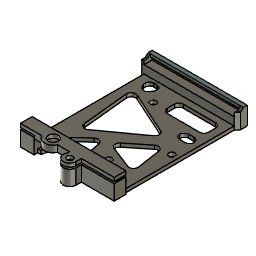
MCU_PCB_mount v14 (Autodesk Fusion 360 design; units mm, degrees)
Autodesk Fusion 360 part; units mm, degrees
sketch "Sketch1" plane through (0, 0, 0) normal (0, 0, 1) x (1, 0, 0)
  line L0 (0, 0) -> (50.2, 0)
  line L1 (50.2, 0) -> (50.2, 70.11)
  line L2 (50.2, 70.11) -> (0, 70.11)
  line L3 (0, 70.11) -> (0, 0)
  dimension "d3" = 50.2
  dimension "d4" = 70.11
  constraint horizontal L0
  constraint vertical L1
  constraint horizontal L2
  constraint vertical L3
  constraint coincident L0.start L3.end
  measures "d3" distance of L1.end L2.end
  measures "d4" distance of L0.end L1.end
extrude "Extrude1" add sketch "Sketch1" along normal blind 2 makes body 1
sketch "holes" plane through (0, 0, 2) normal (0, 0, 1) x (-1, 0, 0)
  line L0 (0, -70.11) -> (0, 0)
  line L1 (0, 0) -> (-50.2, 0)
  line L2 (-50.2, 0) -> (-50.2, -70.11)
  line L3 (-50.2, -70.11) -> (0, -70.11)
  line L4 (-14.9, 0) -> (-14.9, -55.81) construction
  line L5 (-14.9, -55.81) -> (-50.2, -55.81) construction
  line L6 (-48.02, -55.81) -> (-48.02, 0) construction
  line L7 (-16.3, -54.41) -> (-21.3533, -54.41) construction
  line L8 (-21.3533, -54.41) -> (-26.4067, -54.41) construction
  line L9 (-26.4067, -54.41) -> (-31.46, -54.41) construction
  line L10 (-31.46, -54.41) -> (-36.5133, -54.41) construction
  line L11 (-36.5133, -54.41) -> (-41.5667, -54.41) construction
  line L12 (-41.5667, -54.41) -> (-46.62, -54.41) construction
  circle A0 centre (-16.3, -54.41) radius 1.5 construction
  circle A1 centre (-21.3533, -54.41) radius 1.5 construction
  circle A2 centre (-26.4067, -54.41) radius 1.5 construction
  circle A3 centre (-31.46, -54.41) radius 1.5 construction
  circle A4 centre (-36.5133, -54.41) radius 1.5 construction
  circle A5 centre (-41.5667, -54.41) radius 1.5 construction
  circle A6 centre (-46.62, -54.41) radius 1.5 construction
  line L13 (-14.9, -55.81) -> (-17.7, -55.81) construction
  line L14 (-17.7, -55.81) -> (-17.7, -53.01) construction
  line L15 (-17.7, -53.01) -> (-14.9, -53.01) construction
  line L16 (-14.9, -53.01) -> (-14.9, -55.81) construction
  line L17 (-14.9, -55.81) -> (-17.7, -53.01) construction
  line L18 (-17.7, -55.81) -> (-14.9, -53.01) construction
  line L19 (-16.3, -54.41) -> (-14.9, -54.41) construction
  line L20 (-46.62, -54.41) -> (-48.02, -54.41) construction
  circle A7 centre (-16.3, -49.437) radius 1.5 construction
  circle A8 centre (-21.3533, -49.437) radius 1.5 construction
  circle A9 centre (-26.4067, -49.437) radius 1.5 construction
  circle A10 centre (-31.46, -49.437) radius 1.5 construction
  circle A11 centre (-36.5133, -49.437) radius 1.5 construction
  circle A12 centre (-41.5667, -49.437) radius 1.5 construction
  circle A13 centre (-46.62, -49.437) radius 1.5 construction
  circle A14 centre (-16.3, -44.464) radius 1.5 construction
  circle A15 centre (-21.3533, -44.464) radius 1.5 construction
  circle A16 centre (-26.4067, -44.464) radius 1.5 construction
  circle A17 centre (-31.46, -44.464) radius 1.5 construction
  circle A18 centre (-36.5133, -44.464) radius 1.5 construction
  circle A19 centre (-41.5667, -44.464) radius 1.5 construction
  circle A20 centre (-46.62, -44.464) radius 1.5 construction
  circle A21 centre (-16.3, -39.491) radius 1.5 construction
  circle A22 centre (-21.3533, -39.491) radius 1.5 construction
  circle A23 centre (-26.4067, -39.491) radius 1.5 construction
  circle A24 centre (-31.46, -39.491) radius 1.5 construction
  circle A25 centre (-36.5133, -39.491) radius 1.5 construction
  circle A26 centre (-41.5667, -39.491) radius 1.5 construction
  circle A27 centre (-46.62, -39.491) radius 1.5 construction
  circle A28 centre (-16.3, -34.518) radius 1.5 construction
  circle A29 centre (-21.3533, -34.518) radius 1.5 construction
  circle A30 centre (-26.4067, -34.518) radius 1.5 construction
  circle A31 centre (-31.46, -34.518) radius 1.5 construction
  circle A32 centre (-36.5133, -34.518) radius 1.5 construction
  circle A33 centre (-41.5667, -34.518) radius 1.5 construction
  circle A34 centre (-46.62, -34.518) radius 1.5 construction
  circle A35 centre (-16.3, -29.545) radius 1.5 construction
  circle A36 centre (-21.3533, -29.545) radius 1.5 construction
  circle A37 centre (-26.4067, -29.545) radius 1.5 construction
  circle A38 centre (-31.46, -29.545) radius 1.5 construction
  circle A39 centre (-36.5133, -29.545) radius 1.5 construction
  circle A40 centre (-41.5667, -29.545) radius 1.5 construction
  circle A41 centre (-46.62, -29.545) radius 1.5 construction
  circle A42 centre (-16.3, -24.572) radius 1.5 construction
  circle A43 centre (-21.3533, -24.572) radius 1.5 construction
  circle A44 centre (-26.4067, -24.572) radius 1.5 construction
  circle A45 centre (-31.46, -24.572) radius 1.5 construction
  circle A46 centre (-36.5133, -24.572) radius 1.5 construction
  circle A47 centre (-41.5667, -24.572) radius 1.5 construction
  circle A48 centre (-46.62, -24.572) radius 1.5 construction
  circle A49 centre (-16.3, -19.599) radius 1.5 construction
  circle A50 centre (-21.3533, -19.599) radius 1.5 construction
  circle A51 centre (-26.4067, -19.599) radius 1.5 construction
  circle A52 centre (-31.46, -19.599) radius 1.5 construction
  circle A53 centre (-36.5133, -19.599) radius 1.5 construction
  circle A54 centre (-41.5667, -19.599) radius 1.5 construction
  circle A55 centre (-46.62, -19.599) radius 1.5 construction
  circle A56 centre (-16.3, -14.626) radius 1.5 construction
  circle A57 centre (-21.3533, -14.626) radius 1.5 construction
  circle A58 centre (-26.4067, -14.626) radius 1.5 construction
  circle A59 centre (-31.46, -14.626) radius 1.5 construction
  circle A60 centre (-36.5133, -14.626) radius 1.5 construction
  circle A61 centre (-41.5667, -14.626) radius 1.5 construction
  circle A62 centre (-46.62, -14.626) radius 1.5 construction
  circle A63 centre (-16.3, -9.653) radius 1.5 construction
  circle A64 centre (-21.3533, -9.653) radius 1.5 construction
  circle A65 centre (-26.4067, -9.653) radius 1.5 construction
  circle A66 centre (-31.46, -9.653) radius 1.5 construction
  circle A67 centre (-36.5133, -9.653) radius 1.5 construction
  circle A68 centre (-41.5667, -9.653) radius 1.5 construction
  circle A69 centre (-46.62, -9.653) radius 1.5 construction
  circle A70 centre (-16.3, -4.68) radius 1.5 construction
  circle A71 centre (-21.3533, -4.68) radius 1.5 construction
  circle A72 centre (-26.4067, -4.68) radius 1.5 construction
  circle A73 centre (-31.46, -4.68) radius 1.5 construction
  circle A74 centre (-36.5133, -4.68) radius 1.5 construction
  circle A75 centre (-41.5667, -4.68) radius 1.5 construction
  circle A76 centre (-46.62, -4.68) radius 1.5 construction
  line L21 (-14.9, -3.27) -> (-48.02, -3.27) construction
  line L22 (-16.3, -3.27) -> (-16.3, -4.67) construction
  line L23 (-16.3, -54.41) -> (-16.3, -55.81) construction
  point P0 (-16.3, -54.41)
  dimension "d8" = 14.9
  dimension "d9" = 14.3
  dimension "d10" = 2.18
  dimension "d13" = 3
  dimension "d14" = 2.8
  dimension "d15" = 5.0533
  dimension "d18" = 0
  dimension "d19" = 49.73
  dimension "d40" = 52.54
  constraint coincident L1 L4.start
  constraint perpendicular L1 L4
  constraint coincident L2 L5.end
  constraint perpendicular L2 L5
  constraint coincident L5 L6.start
  constraint coincident L1 L6.end
  constraint perpendicular L1 L6
  constraint perpendicular L4 L7
  constraint perpendicular L4 L8
  constraint parallel L8 L9
  constraint parallel L9 L10
  constraint parallel L10 L11
  constraint parallel L11 L12
  constraint equal L7 L8
  constraint equal L8 L9
  constraint equal L9 L10
  constraint equal L10 L11
  constraint equal L11 L12
  constraint coincident P0 L7.start
  constraint coincident L7.end L8.start
  constraint coincident L8.end L9.start
  constraint coincident L9.end L10.start
  constraint coincident L10.end L11.start
  constraint coincident L11.end L12.start
  constraint coincident L12.end A6.centre
  constraint equal A0 A1
  constraint equal A1 A2
  constraint equal A2 A3
  constraint equal A3 A4
  constraint equal A4 A5
  constraint equal A5 A6
  constraint horizontal L13
  constraint perpendicular L13 L14
  constraint parallel L13 L15
  constraint parallel L14 L16
  constraint coincident L17 P0
  constraint coincident L18 P0
  constraint equal L14 L15
  constraint midpoint L16 L19.end
  constraint coincident L6 L20.end
  constraint perpendicular L6 L20
  constraint equal L19 L20
  constraint coincident L4 L21.start
  constraint coincident L6 L21.end
  constraint perpendicular L6 L21
  constraint coincident L21 L22.start
  constraint perpendicular L21 L22
  constraint midpoint L13 L23.end
  constraint equal L22 L23
  constraint vertical A70.centre L22.end
  measures "d8" distance of L0 L4
  measures "d9" distance of L3 L5
  measures "d10" distance of L2 L6
  measures "d13" diameter of A0
  measures "d14" distance of L13.end L14.end
  measures "d15" distance of P0 L7.end
  measures "d40" distance of L5 L21
sketch "screw-around" plane through (0, 0, 2) normal (0, 0, 1) x (-1, 0, 0)
  line L0 (0, -70.11) -> (0, 0)
  line L1 (0, 0) -> (-50.2, 0)
  line L2 (-50.2, 0) -> (-50.2, -70.11)
  line L3 (-50.2, -70.11) -> (0, -70.11)
  line L4 (-15.1, -3.845) -> (-15.1, 3.845) construction
  circle A0 centre (-15.1, 0) radius 3.845 construction
  dimension "d68" = 15.1
  dimension "d69" = 7.69
  constraint perpendicular L1 L4
  constraint coincident L4 A0.centre
  constraint coincident L1 A0.centre
  constraint coincident L4.start A0
  constraint coincident L4.end A0
  measures "d68" distance of L0 L4
  measures "d69" diameter of A0
sketch "Sketch7" plane through (0, 0, 2) normal (0, 0, 1) x (-1, 0, 0)
  line L0 (0, -70.11) -> (0, 0)
  line L1 (0, 0) -> (-50.2, 0)
  line L2 (-50.2, 0) -> (-50.2, -70.11)
  line L3 (-50.2, -70.11) -> (0, -70.11)
  circle A0 centre (-16.3, -54.41) radius 1.5
  circle A1 centre (-31.46, -4.68) radius 1.5
  circle A2 centre (-46.62, -34.518) radius 1.5
  circle A3 centre (-31.46, -14.626) radius 1.5
extrude "Extrude6" cut sketch "Sketch7" against normal up to surface (2 mm away) contours A0 | A2 | A3 bodies 1
sketch "Sketch8" plane through (0, 0, 0) normal (0, 0, 1) x (1, 0, 0)
  line L0 (-1.6, 65.61) -> (51.8, 65.61)
  line L1 (51.8, 65.61) -> (51.8, 71.71)
  line L2 (51.8, 71.71) -> (-1.6, 71.71)
  line L3 (-1.6, 71.71) -> (-1.6, 65.61)
  line L4 (50.2, 70.11) -> (0, 70.11)
  line L5 (0, 70.11) -> (0, 0) construction
  line L6 (50.2, 0) -> (50.2, 70.11) construction
  dimension "d45" = 4.5
  dimension "d46" = 1.6
  dimension "d47" = 1.6
  dimension "d48" = 1.6
  constraint horizontal L0
  constraint vertical L1
  constraint horizontal L2
  constraint vertical L3
  measures "d45" distance of L0 L4
  measures "d46" distance of L2 L4
  measures "d47" distance of L3 L5
  measures "d48" distance of L1 L6
extrude "Extrude7" add sketch "Sketch8" along normal blind 6.5 bodies 1
sketch "Sketch9" plane through (0, 0, 6.5) normal (0, 0, 1) x (-1, 0, 0)
  line L0 (1.6, -71.71) -> (1.6, -65.61)
  line L1 (1.6, -65.61) -> (-51.8, -65.61)
  line L2 (-51.8, -65.61) -> (-51.8, -71.71)
  line L3 (-51.8, -71.71) -> (1.6, -71.71)
  line L4 (0, -65.61) -> (-50.2, -65.61)
  line L5 (-50.2, -65.61) -> (-50.2, -70.11)
  line L6 (-50.2, -70.11) -> (0, -70.11)
  line L7 (0, -70.11) -> (0, -65.61)
  line L8 (0, -65.61) -> (0, 0)
  line L9 (-50.2, 0) -> (-50.2, -65.61)
  dimension "d51" = 1.6
  constraint horizontal L4
  constraint vertical L5
  constraint horizontal L6
  constraint vertical L7
  constraint coincident L1 L4.start
  constraint collinear L7 L8
  constraint collinear L5 L9
  measures "d51" distance of L3 L6
extrude "Extrude8" add sketch "Sketch9" along normal blind 1.9 contours L0 L1 L2 L3 L5 L6 L7 bodies 1
sketch "Sketch10" plane through (0, 0, 8.4) normal (0, 0, 1) x (-1, 0, 0)
  line L0 (-50.2, -65.61) -> (-51.8, -65.61)
  line L1 (-51.8, -65.61) -> (-51.8, -71.71)
  line L2 (-51.8, -71.71) -> (1.6, -71.71)
  line L3 (1.6, -71.71) -> (1.6, -65.61)
  line L4 (1.6, -65.61) -> (0, -65.61)
  line L5 (0, -65.61) -> (0, -70.11)
  line L6 (0, -70.11) -> (-50.2, -70.11)
  line L7 (-50.2, -70.11) -> (-50.2, -65.61)
  line L8 (1.6, -71.71) -> (-51.8, -71.71)
  line L9 (-51.8, -71.71) -> (-51.8, -69.11)
  line L10 (-51.8, -69.11) -> (1.6, -69.11)
  line L11 (1.6, -69.11) -> (1.6, -71.71)
  dimension "d56" = 1
  constraint horizontal L8
  constraint vertical L9
  constraint horizontal L10
  constraint vertical L11
  constraint coincident L1 L9.end
  constraint coincident L2.end L3.start
  measures "d56" distance of L6 L10
extrude "Extrude9" add sketch "Sketch10" along normal blind 1.6 contours L5 L6 L7 L10 | L1 L2 L3 L5 L6 L7 L8 L9 L10 L11 bodies 1
chamfer "Chamfer1" distance 1.6 angle 45 2 edges at (-0.8, 69.11, 8.4) (51, 69.11, 8.4) on bodies 1
sketch "Sketch11" plane through (0, 0, 0) normal (0, 0, 1) x (1, 0, 0)
  line L0 (-1.6, 4.5) -> (51.8, 4.5)
  line L1 (51.8, 4.5) -> (51.8, -2)
  line L2 (51.8, -2) -> (-1.6, -2)
  line L3 (-1.6, -2) -> (-1.6, 4.5)
  line L4 (0, 0) -> (50.2, 0)
  line L5 (6.4, 4.5) -> (6.4, -2)
  line L6 (27.8, 4.5) -> (27.8, -2)
  point P0 (-1.6, 65.61)
  point P1 (51.8, 65.61)
  dimension "d60" = 2
  dimension "d61" = 4.5
  dimension "d62" = 24
  dimension "d63" = 8
  constraint horizontal L0
  constraint vertical L1
  constraint horizontal L2
  constraint vertical L3
  constraint vertical L0.start P0
  constraint vertical L0.end P1
  constraint coincident L0 L5.start
  constraint coincident L2 L5.end
  constraint perpendicular L2 L5
  constraint coincident L0 L6.start
  constraint coincident L2 L6.end
  constraint perpendicular L2 L6
  measures "d60" distance of L2 L4
  measures "d61" distance of L0 L4
  measures "d62" distance of L1 L6
  measures "d63" distance of L3 L5
extrude "Extrude10" add sketch "Sketch11" along normal up to surface (8.4 mm away) contours L0 L2 L3 L5 | L0 L1 L2 L6 bodies 1
sketch "Sketch12" plane through (0, 0, 8.4) normal (0, 0, 1) x (-1, 0, 0)
  line L0 (-6.4, 2) -> (-6.4, -4.5)
  line L1 (-6.4, -4.5) -> (1.6, -4.5)
  line L2 (1.6, -4.5) -> (1.6, 2)
  line L3 (1.6, 2) -> (-6.4, 2)
  line L4 (0, 0.4) -> (-50.2, 0.4)
  line L5 (-50.2, 0.4) -> (-50.2, -4.5)
  line L6 (-50.2, -4.5) -> (0, -4.5)
  line L7 (0, -4.5) -> (0, 0.4)
  line L8 (-50.2, -4.5) -> (-50.2, -65.61)
  line L9 (0, -65.61) -> (0, -4.5)
  line L10 (-6.4, 0) -> (-27.8, 0) construction
  dimension "d80" = 0.4
  constraint horizontal L4
  constraint vertical L5
  constraint horizontal L6
  constraint vertical L7
  constraint collinear L5 L8
  constraint collinear L1 L6
  constraint coincident L4.end L5.start
  constraint collinear L7 L9
  measures "d80" distance of L4 L10
extrude "Extrude11" cut sketch "Sketch12" against normal up to surface (1.9 mm away) contours L0 L1 L4 L6 L7 | L0 L4 L5 L6 bodies 1
sketch "Sketch14" plane through (0, 0, 2) normal (0, 0, 1) x (-1, 0, 0)
  line L0 (-27.8, -4.5) -> (-50.2, -4.5)
  line L1 (-50.2, -4.5) -> (-50.2, -65.61)
  line L2 (-50.2, -65.61) -> (0, -65.61)
  line L3 (0, -65.61) -> (0, -4.5)
  line L4 (0, -4.5) -> (-6.4, -4.5)
  line L5 (-6.4, -4.5) -> (-6.4, 0)
  line L6 (-6.4, 0) -> (-27.8, 0)
  line L7 (-27.8, 0) -> (-27.8, -4.5)
  circle A0 centre (-16.3, -54.41) radius 1.5
  circle A1 centre (-46.62, -34.518) radius 1.5
  circle A2 centre (-31.46, -14.626) radius 1.5
  circle A3 centre (-15.1, 0) radius 3.845 construction
  circle A4 centre (-15.1, 0) radius 6.845
  dimension "d70" = 3
  constraint concentric A3 A4
  measures "d70" distance of A3 A4
extrude "Extrude12" cut sketch "Sketch14" against normal up to surface (2 mm away) contours L6 A4 picked at (-15.9336, -2.8041) bodies 1
sketch "Sketch15" plane through (0, 0, 0) normal (0, 0, 1) x (1, 0, 0)
  circle A0 centre (29.2, -5) radius 1.5
  circle A1 centre (29.2, -5) radius 3.5
  line L0 (21.945, 0) -> (27.8, 0)
  line L1 (50.2, 4.5) -> (50.2, -0.4)
  line L2 (32.7, -5) -> (32.7, -0.4)
  line L3 (26.1623, -3.2615) -> (27.8, -0.4)
  line L4 (27.8, -0.4) -> (32.7, -0.4)
  point P0 (27.8, -0.4)
  dimension "d73" = 3
  dimension "d74" = 2
  dimension "d76" = 5
  dimension "d77" = 21
  constraint concentric A0 A1
  constraint coincident A1 L2.start
  constraint perpendicular L0 L2
  constraint tangent A1 L2
  constraint coincident A1 L3.start
  constraint coincident P0 L3.end
  constraint tangent A1 L3
  constraint perpendicular L2 L4
  measures "d73" diameter of A0
  measures "d74" distance of A0 A1
  measures "d76" distance of A0.centre L0
  measures "d77" distance of A0.centre L1
extrude "Extrude13" add sketch "Sketch15" along normal up to surface (8.4 mm away) bodies 1
fillet "Fillet1" radius 15.75 1 edges at (27.8, -0.4, 3.25) on bodies 1
fillet "Fillet2" radius 2 1 edges at (27.3488, 0, 1) on bodies 1
sketch "cuts" plane through (0, 0, 2) normal (0, 0, 1) x (-1, 0, 0)
  arc A0 (-26.3604, 2.8353) -> (-27.8, -3.743) centre (-12.05, -3.743) ccw
  line L0 (-27.8, -3.743) -> (-27.8, -4.5)
  line L1 (-27.8, -4.5) -> (-50.2, -4.5)
  line L2 (-50.2, -4.5) -> (-50.2, -65.61)
  line L3 (-50.2, -65.61) -> (0, -65.61)
  line L4 (0, -65.61) -> (0, -4.5)
  line L5 (0, -4.5) -> (-6.4, -4.5)
  line L6 (-6.4, -4.5) -> (-6.4, 0)
  line L7 (-6.4, 0) -> (-8.255, 0)
  arc A1 (-21.945, 0) -> (-8.255, 0) centre (-15.1, 0) ccw
  line L8 (-21.945, 0) -> (-24.5432, 0)
  arc A2 (-26.3604, 2.8353) -> (-24.5432, 0) centre (-24.5432, 2) ccw
  circle A3 centre (-16.3, -54.41) radius 1.5
  circle A4 centre (-46.62, -34.518) radius 1.5
  circle A5 centre (-31.46, -14.626) radius 1.5
  line L9 (-36, -41) -> (-4.2679, -55.3205)
  line L10 (-4.2679, -55.3205) -> (-7.7321, -20.6795)
  line L11 (-7.7321, -20.6795) -> (-36, -41)
  line L12 (-44, -15) -> (-40.6603, -36.9282)
  line L13 (-40.6603, -36.9282) -> (-23.3397, -23.0718)
  line L14 (-23.3397, -23.0718) -> (-44, -15)
  line L15 (-23, -62) -> (-46, -62)
  line L16 (-46, -62) -> (-46, -53)
  line L17 (-46, -53) -> (-23, -53)
  line L18 (-23, -53) -> (-23, -62)
  line L19 (-39, -49) -> (-47, -49)
  line L20 (-47, -49) -> (-47, -44)
  line L21 (-47, -44) -> (-39, -44)
  line L22 (-39, -44) -> (-39, -49)
  line L23 (-37, -10) -> (-47, -10)
  line L24 (-47, -10) -> (-47, -6)
  line L25 (-47, -6) -> (-37, -6)
  line L26 (-37, -6) -> (-37, -10)
  line L27 (-20.2679, -23.6603) -> (-7, -12)
  line L28 (-7, -12) -> (-23.7321, -6.3397)
  line L29 (-23.7321, -6.3397) -> (-20.2679, -23.6603)
  line L30 (-2.8038, -64) -> (-8, -55)
  line L31 (-8, -55) -> (-13.1962, -64)
  line L32 (-13.1962, -64) -> (-2.8038, -64)
  point P0 (-16, -39)
  point P1 (-36, -25)
  point P2 (-17, -14)
  point P3 (-8, -61)
  constraint horizontal L15
  constraint vertical L16
  constraint horizontal L17
  constraint vertical L18
  constraint horizontal L19
  constraint vertical L20
  constraint horizontal L21
  constraint vertical L22
  constraint horizontal L23
  constraint vertical L24
  constraint horizontal L25
  constraint vertical L26
extrude "cuts" cut sketch "cuts" against normal up to surface (2 mm away) contours L9 L10 L11 | L12 L13 L14 | L15 L16 L17 L18 | L19 L20 L21 L22 | L23 L24 L25 L26 | L27 L28 L29 | L30 L31 L32 bodies 1
fillet "Fillet3" radius 2.5 24 edges at (36, 41, 1) (4.2679, 55.3205, 1) (7.7321, 20.6795, 1) (7, 12, 1) (20.2679, 23.6603, 1) (40.6603, 36.9282, 1) (47, 49, 1) (46, 62, 1) (23.7321, 6.3397, 1) (44, 15, 1) (47, 6, 1) (23.3397, 23.0718, 1) (37, 6, 1) (39, 44, 1) (23, 53, 1) (37, 10, 1) (47, 10, 1) (39, 49, 1) (23, 62, 1) (2.8038, 64, 1) (13.1962, 64, 1) (46, 53, 1) (47, 44, 1) (8, 55, 1) on bodies 1
ref_plane "WorkPlane1" through (38.3733, -2.3137, 9.4) normal (0, 0, 1) x (1, 0, 0)
sketch "Sketch17" plane through (38.5752, -2.3138, 9.4) normal (0, 0, 1) x (1, 0, 0)
  arc A0 (-12.4933, -1.0965) -> (-5.8752, -2.6862) centre (-9.3752, -2.6862) ccw construction
  line L0 (-10.7752, 6.8138) -> (11.6248, 6.8138) construction
  line L1 (13.2248, 6.8138) -> (13.2248, 0.3138) construction
  line L2 (-40.1752, 0.3138) -> (-40.1752, 6.8138) construction
  line L3 (13.2248, 0.3138) -> (-5.8752, 0.3138) construction
  circle A1 centre (-23.4752, 2.3138) radius 3.845 construction
  circle A2 centre (-9.3752, -2.6862) radius 3.5
  circle A3 centre (-9.3752, -2.6862) radius 1.7
  line L4 (-5.8752, -2.6862) -> (-5.8752, 0.3138)
  line L5 (-5.8752, 0.3138) -> (13.2248, 0.3138)
  line L6 (13.2248, 0.3138) -> (13.2248, 6.8138)
  line L7 (13.2248, 6.8138) -> (-40.1752, 6.8138)
  line L8 (-40.1752, 6.8138) -> (-40.1752, 0.3138)
  line L9 (-40.1752, 0.3138) -> (-27.8386, 0.3138)
  line L10 (-12.4933, -1.0965) -> (-12.4933, 0.3138)
  line L11 (-12.4933, 0.3138) -> (-19.1117, 0.3138)
  arc A4 (-27.8386, 0.3138) -> (-19.1117, 0.3138) centre (-23.4752, 2.3138) ccw
  circle A5 centre (-23.4752, 2.3138) radius 2.8
  dimension "d90" = 3.4
  dimension "d93" = 5.6
  dimension "d94" = 2
  constraint concentric A0 A2
  constraint coincident A0.end A2
  constraint concentric A0 A3
  constraint coincident A0.end L4.start
  constraint coincident L3.end L4.end
  constraint coincident L1.end L3.start
  constraint coincident L1.start L6.end
  constraint coincident L2.end L7.end
  constraint coincident L2.start L8.end
  constraint perpendicular L8 L9
  constraint coincident A0.start L10.start
  constraint vertical L10
  constraint perpendicular L10 L11
  constraint coincident A1.centre A4.centre
  constraint coincident L9.end A4.start
  constraint collinear L9 L11
  constraint concentric A4 A5
  measures "d90" diameter of A3
  measures "d93" diameter of A5
  measures "d94" distance of A4 A5
extrude "Extrude15" add sketch "Sketch17" along normal blind 2 separate body makes body 2
sketch "Sketch18" plane through (0, 0, 9.4) normal (0, 0, -1) x (1, 0, 0)
  circle A0 centre (29.2, 5) radius 1.7
  circle A1 centre (15.1, 0) radius 2.8
  arc A2 (32.7, 5) -> (26.0818, 3.4104) centre (29.2, 5) ccw
  line L0 (26.0818, 3.4104) -> (26.0818, 2)
  line L1 (26.0818, 2) -> (19.4635, 2)
  arc A3 (19.4635, 2) -> (10.7365, 2) centre (15.1, 0) ccw
  line L2 (10.7365, 2) -> (-1.6, 2)
  line L3 (-1.6, 2) -> (-1.6, -4.5)
  line L4 (-1.6, -4.5) -> (51.8, -4.5)
  line L5 (51.8, -4.5) -> (51.8, 2)
  line L6 (51.8, 2) -> (32.7, 2)
  line L7 (32.7, 2) -> (32.7, 5)
  line L8 (6.4, 0.4) -> (6.4, 2) construction
  arc A4 (27.2453, 0.4) -> (26.0818, 3.4104) centre (12.05, -3.743) ccw construction
  line L9 (26.0818, 2) -> (26.0818, 0.4)
  line L10 (26.0818, 0.4) -> (17.8713, 0.4)
  line L11 (6.8, 2) -> (6.8, 0.4)
  line L12 (6.8, 0.4) -> (12.3287, 0.4)
  line L13 (10.7365, 2) -> (19.4635, 2)
  circle A5 centre (15.1, 0) radius 2.8 construction
  arc A6 (13.6578, 2.4) -> (12.3287, 0.4) centre (15.1, 0) ccw
  arc A7 (17.8713, 0.4) -> (17.0596, 2) centre (15.1, 0) ccw
  dimension "d97" = 0.4
  constraint coincident L0.end L1.start
  constraint perpendicular L1 L9
  constraint coincident A1 L10.end
  constraint perpendicular L9 L10
  constraint coincident L2 L11.start
  constraint perpendicular L2 L11
  constraint coincident A1 L12.end
  constraint perpendicular L11 L12
  constraint collinear L10 L12
  constraint horizontal L8.start L11.end
  constraint coincident A3.end L2.start
  constraint coincident L1.end A3.start
  constraint equal A1 A5
  constraint concentric A1 A5
  constraint coincident A1.centre A3.centre
  constraint coincident A5 A7.end
  constraint coincident L13 A7.end
  measures "d97" distance of L8 L11
extrude "Extrude16" add sketch "Sketch18" along normal blind 1.7 contours A1 L1 L9 L10 L13 A7 | A1 L2 L11 L12 L13 A6 | A1 A3 L13 A6 bodies 2
sketch "Sketch19" plane through (0, 0, 2) normal (0, 0, 1) x (-1, 0, 0)
  line L0 (-39.9668, -16.5758) -> (-27.373, -21.496)
  arc A0 (-26.721, -25.7768) -> (-27.373, -21.496) centre (-28.2827, -23.8246) ccw
  line L1 (-26.721, -25.7768) -> (-37.279, -34.2232)
  arc A1 (-41.3122, -32.6474) -> (-37.279, -34.2232) centre (-38.8407, -32.271) ccw
  line L2 (-41.3122, -32.6474) -> (-43.348, -19.2808)
  arc A2 (-39.9668, -16.5758) -> (-43.348, -19.2808) centre (-40.8765, -18.9043) ccw
  line L3 (-32.484, -38.4725) -> (-11.248, -23.2069)
  arc A3 (-7.3012, -24.9881) -> (-11.248, -23.2069) centre (-9.7888, -25.2369) ccw
  line L4 (-7.3012, -24.9881) -> (-4.6988, -51.0119)
  arc A4 (-8.2148, -53.5393) -> (-4.6988, -51.0119) centre (-7.1864, -51.2606) ccw
  line L5 (-8.2148, -53.5393) -> (-32.0532, -42.7812)
  arc A5 (-32.484, -38.4725) -> (-32.0532, -42.7812) centre (-31.0248, -40.5025) ccw
  line L6 (-44.5, -44) -> (-41.5, -44)
  arc A6 (-39, -46.5) -> (-41.5, -44) centre (-41.5, -46.5) ccw
  arc A7 (-41.5, -49) -> (-39, -46.5) centre (-41.5, -46.5) ccw
  line L7 (-41.5, -49) -> (-44.5, -49)
  arc A8 (-47, -46.5) -> (-44.5, -49) centre (-44.5, -46.5) ccw
  arc A9 (-44.5, -44) -> (-47, -46.5) centre (-44.5, -46.5) ccw
  line L8 (-44.5, -6) -> (-39.5, -6)
  arc A10 (-37, -8.5) -> (-39.5, -6) centre (-39.5, -8.5) ccw
  arc A11 (-39.2913, -10) -> (-37, -8.5) centre (-39.2913, -7.5) ccw
  line L9 (-39.2913, -10) -> (-44.7087, -10)
  arc A12 (-47, -8.5) -> (-44.7087, -10) centre (-44.7087, -7.5) ccw
  arc A13 (-44.5, -6) -> (-47, -8.5) centre (-44.5, -8.5) ccw
  line L10 (-7.134, -64) -> (-8.866, -64)
  arc A14 (-11.0311, -60.25) -> (-8.866, -64) centre (-8.866, -61.5) ccw
  line L11 (-11.0311, -60.25) -> (-10.1651, -58.75)
  arc A15 (-5.8349, -58.75) -> (-10.1651, -58.75) centre (-8, -60) ccw
  line L12 (-5.8349, -58.75) -> (-4.9689, -60.25)
  arc A16 (-7.134, -64) -> (-4.9689, -60.25) centre (-7.134, -61.5) ccw
  line L13 (-43.5, -53) -> (-25.5, -53)
  arc A17 (-23, -55.5) -> (-25.5, -53) centre (-25.5, -55.5) ccw
  line L14 (-23, -55.5) -> (-23, -59.5)
  arc A18 (-25.5, -62) -> (-23, -59.5) centre (-25.5, -59.5) ccw
  line L15 (-25.5, -62) -> (-43.5, -62)
  arc A19 (-46, -59.5) -> (-43.5, -62) centre (-43.5, -59.5) ccw
  line L16 (-46, -59.5) -> (-46, -55.5)
  arc A20 (-43.5, -53) -> (-46, -55.5) centre (-43.5, -55.5) ccw
  line L17 (-21.1172, -19.4142) -> (-22.8828, -10.5858)
  arc A21 (-19.6303, -7.7273) -> (-22.8828, -10.5858) centre (-20.4314, -10.0955) ccw
  line L18 (-19.6303, -7.7273) -> (-11.1018, -10.6124)
  arc A22 (-10.2526, -14.8585) -> (-11.1018, -10.6124) centre (-11.9029, -12.9806) ccw
  line L19 (-10.2526, -14.8585) -> (-17.0154, -20.8018)
  arc A23 (-21.1172, -19.4142) -> (-17.0154, -20.8018) centre (-18.6657, -18.9239) ccw
  arc A24 (-26.3604, 2.8353) -> (-27.8, -3.743) centre (-12.05, -3.743) ccw
  line L20 (-27.8, -3.743) -> (-27.8, -4.5)
  line L21 (-27.8, -4.5) -> (-50.2, -4.5)
  line L22 (-50.2, -4.5) -> (-50.2, -65.61)
  line L23 (-50.2, -65.61) -> (0, -65.61)
  line L24 (0, -65.61) -> (0, -4.5)
  line L25 (0, -4.5) -> (-6.4, -4.5)
  line L26 (-6.4, -4.5) -> (-6.4, 0)
  line L27 (-6.4, 0) -> (-8.255, 0)
  arc A25 (-21.945, 0) -> (-8.255, 0) centre (-15.1, 0) ccw
  line L28 (-21.945, 0) -> (-24.5432, 0)
  arc A26 (-26.3604, 2.8353) -> (-24.5432, 0) centre (-24.5432, 2) ccw
  circle A27 centre (-16.3, -54.41) radius 1.5
  circle A28 centre (-46.62, -34.518) radius 1.5
  circle A29 centre (-31.46, -14.626) radius 1.5
  circle A30 centre (-16.3, -54.41) radius 1.7
  circle A31 centre (-46.62, -34.518) radius 1.7
  circle A32 centre (-31.46, -14.626) radius 1.7
  dimension "d100" = 3.4
  constraint concentric A27 A30
  constraint concentric A28 A31
  constraint concentric A29 A32
  constraint equal A30 A31
  constraint equal A31 A32
  measures "d100" diameter of A30
extrude "Extrude17" cut sketch "Sketch19" against normal up to surface (2 mm away) contours A30 | A31 | A32 bodies 1
sketch "Sketch20" plane through (0, 0, 11.4) normal (0, 0, 1) x (-1, 0, 0)
  circle A0 centre (-29.2, 5) radius 1.7
  circle A1 centre (-15.1, 0) radius 2.8
  arc A2 (-26.0818, 3.4104) -> (-32.7, 5) centre (-29.2, 5) ccw
  line L0 (-32.7, 5) -> (-32.7, 2)
  line L1 (-32.7, 2) -> (-51.8, 2)
  line L2 (-51.8, 2) -> (-51.8, -4.5)
  line L3 (-51.8, -4.5) -> (1.6, -4.5)
  line L4 (1.6, -4.5) -> (1.6, 2)
  line L5 (1.6, 2) -> (-10.7365, 2)
  arc A3 (-10.7365, 2) -> (-19.4635, 2) centre (-15.1, 0) ccw
  line L6 (-19.4635, 2) -> (-26.0818, 2)
  line L7 (-26.0818, 2) -> (-26.0818, 3.4104)
  line L8 (-51.8, -4.5) -> (-51, -4.5)
  line L9 (-51, -4.5) -> (-51, 2)
  line L10 (-51, 2) -> (-51.8, 2)
  line L11 (-51.8, 2) -> (-51.8, -4.5)
  line L12 (-50.2, -4.5) -> (-50.2, -65.61) construction
  dimension "d103" = 0.8
  constraint horizontal L8
  constraint vertical L9
  constraint horizontal L10
  constraint vertical L11
  constraint coincident L1 L9.end
  constraint coincident L2.end L3.start
  measures "d103" distance of L9 L12
extrude "Extrude18" cut sketch "Sketch20" against normal up to surface (11.4 mm away) contours L1 L2 L3 L8 L9 L10 L11 bodies 1 2
sketch "Sketch21" plane through (0, 0, 8.4) normal (0, 0, 1) x (-1, 0, 0)
  line L0 (-51.8, -67.51) -> (-50.2, -67.51)
  line L1 (-50.2, -67.51) -> (-50.2, -65.61)
  line L2 (-50.2, -65.61) -> (-51.8, -65.61)
  line L3 (-51.8, -65.61) -> (-51.8, -67.51)
  line L4 (-51.8, -65.61) -> (-51.8, -67.51)
  line L5 (-51.8, -67.51) -> (-50.2, -65.61)
  line L6 (-51.8, -65.61) -> (-50.2, -65.61)
  constraint coincident L2.end L3.start
  constraint perpendicular L2 L4
  constraint coincident L0.start L3.end
  constraint coincident L1.end L2.start
extrude "Extrude19" cut sketch "Sketch21" against normal up to surface (8.4 mm away) contours L2 L3 L4 L5 L6 bodies 1
sketch "Sketch22" plane through (0, 0, 10) normal (0, 0, 1) x (-1, 0, 0)
  line L0 (1.6, -69.11) -> (0, -69.11)
  line L1 (0, -69.11) -> (-50.2, -69.11)
  line L2 (-50.2, -69.11) -> (-51.8, -69.11)
  line L3 (-51.8, -69.11) -> (-51.8, -71.71)
  line L4 (-51.8, -71.71) -> (1.6, -71.71)
  line L5 (1.6, -71.71) -> (1.6, -69.11)
  line L6 (1.6, -71.71) -> (-51.8, -71.71)
  line L7 (-51.8, -71.71) -> (-51.8, -71.31)
  line L8 (-51.8, -71.31) -> (1.6, -71.31)
  line L9 (1.6, -71.31) -> (1.6, -71.71)
  dimension "d108" = 0.4
  constraint horizontal L6
  constraint vertical L7
  constraint horizontal L8
  constraint vertical L9
  constraint coincident L3 L7.end
  constraint coincident L4.end L5.start
  measures "d108" distance of L6 L8
extrude "Extrude20" cut sketch "Sketch22" against normal up to surface (10 mm away) contours L3 L4 L5 L6 L7 L8 L9 bodies 1
sketch "Sketch23" plane through (0, 0, 11.4) normal (0, 0, 1) x (-1, 0, 0)
  line L0 (-51, 2) -> (-51, -4.5)
  line L1 (-51, -4.5) -> (1.6, -4.5)
  line L2 (1.6, -4.5) -> (1.6, 2)
  line L3 (1.6, 2) -> (-10.7365, 2)
  arc A0 (-10.7365, 2) -> (-19.4635, 2) centre (-15.1, 0) ccw
  line L4 (-19.4635, 2) -> (-26.0818, 2)
  line L5 (-26.0818, 2) -> (-26.0818, 3.4104)
  arc A1 (-26.0818, 3.4104) -> (-32.7, 5) centre (-29.2, 5) ccw
  line L6 (-32.7, 5) -> (-32.7, 2)
  line L7 (-32.7, 2) -> (-51, 2)
  circle A2 centre (-29.2, 5) radius 1.7
  circle A3 centre (-15.1, 0) radius 2.8
  line L8 (1.2, -4.5) -> (1.2, 2)
  line L9 (1.2, -4.5) -> (1.2, -85)
  line L10 (-51.8, -71.31) -> (1.6, -71.31)
  line L11 (1.6, -71.31) -> (1.6, -69.11)
  line L12 (1.6, -69.11) -> (1.6, -67.51)
  line L13 (1.6, -67.51) -> (1.6, -65.61)
  line L14 (1.6, -65.61) -> (0, -65.61)
  dimension "d111" = 0.4
  constraint coincident L1 L8.start
  constraint coincident L3 L8.end
  constraint perpendicular L3 L8
  constraint perpendicular L1 L9
  measures "d111" distance of L2 L8
extrude "Extrude21" cut sketch "Sketch23" against normal blind 22 contours L1 L2 L3 L8 | L9 L10 L11 L12 L13 L14 bodies 1 2
sketch "Sketch24" plane through (0, 0, 10) normal (0, 0, 1) x (-1, 0, 0)
  line L0 (1.2, -71.31) -> (1.2, -69.11)
  line L1 (1.2, -69.11) -> (0, -69.11)
  line L2 (0, -69.11) -> (-50.2, -69.11)
  line L3 (-50.2, -69.11) -> (-51.8, -69.11)
  line L4 (-51.8, -69.11) -> (-51.8, -71.31)
  line L5 (-51.8, -71.31) -> (1.2, -71.31)
equation "board_L = 70.11 mm"
equation "board_W = 50.2 mm"
equation "d3 = board_W"
equation "d4 = board_L"
equation "bottom_t = 2 mm" comment "change to 2 after testing"
equation "d6 = bottom_t"
equation "M3_D = 3 mm"
equation "d13 = M3_D"
equation "d19 = 50.53 mm - 1.4 mm + 0.6 mm"
equation "standoff_H = 4.5 mm"
equation "wall_t = 1.6 mm"
equation "d46 = wall_t"
equation "d47 = wall_t"
equation "d48 = wall_t"
equation "d49 = bottom_t + standoff_H"
equation "d51 = wall_t"
equation "pcb_t = 1.5 mm"
equation "clearance = 0.2 mm"
equation "d54 = pcb_t + clearance * 2"
equation "d57 = wall_t"
equation "d60 = wall_t + clearance * 2"
equation "d73 = M3_D"
equation "screwhole_space_d = 5 mm"
equation "d76 = screwhole_space_d"
equation "d80 = clearance * 2"
equation "d90 = M3_D + clearance * 2"
equation "screwg_D = 4.8 mm"
equation "d93 = screwg_D + clearance * 4"
equation "d95 = bottom_t"
equation "d97 = clearance * 2"
equation "d98 = pcb_t + clearance"
equation "d100 = M3_D + clearance * 2"
